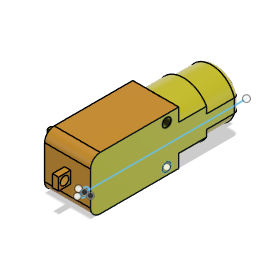
Moto-réducteur (Autodesk Fusion 360 design; units mm, degrees)
Autodesk Fusion 360 part; units mm, degrees
note: some values were not read from the file. Set by a fixed rule: which sketch regions a step uses.
sketch "Sketch1" plane through (0, 0, 0) normal (0, 0, 1) x (1, 0, 0)
  line L0 (0, 0) -> (19, 0)
  line L1 (19, 0) -> (19, 22)
  line L2 (19, 22) -> (0, 22)
  line L3 (0, 22) -> (0, 0)
  line L4 (0, 22) -> (19, 0)
  line L5 (19, 22) -> (0, 0)
  arc A0 (0, 5.4547) -> (19, 5.4547) centre (9.5, 11) ccw
  arc A1 (19, 16.5453) -> (0, 16.5453) centre (9.5, 11) ccw
  dimension "d1" = 19
  dimension "d2" = 22
  constraint horizontal L0
  constraint vertical L1
  constraint horizontal L2
  constraint vertical L3
  constraint coincident L0.start L3.end
  constraint midpoint L4 A0.centre
  constraint tangent L2 A0
  constraint coincident L3 A1.end
  constraint coincident L3 A0.start
  constraint coincident L1 A0.end
  constraint coincident L1 A1.start
  constraint concentric A0 A1
  measures "d1" distance of L0.start L0.end
  measures "d2" distance of L0.start L2.end
extrude "Extrude1" add sketch "Sketch1" along normal blind 36.5
extrude "Extrude2" add sketch "Sketch1" against normal blind 11.5 contours L4 L5 A0 | L3 L4 L5 A0 A1 | L1 L4 L5 A0 A1 | L4 L5 A1
sketch "Sketch2" plane through (0, 0, -11.5) normal (0, 0, -1) x (-1, 0, 0)
  arc A0 (0, 16.5453) -> (-19, 16.5453) centre (-9.5, 11) ccw
  line L0 (-19, 16.5453) -> (-19, 5.4547)
  arc A1 (-19, 5.4547) -> (0, 5.4547) centre (-9.5, 11) ccw
  line L1 (0, 5.4547) -> (0, 16.5453)
  arc A2 (-19, 8.2143) -> (0, 8.2143) centre (-9.5, 11) ccw
  arc A3 (0, 13.7857) -> (-19, 13.7857) centre (-9.5, 11) ccw
  line L2 (-19, 13.7857) -> (-19, 8.2143)
  line L3 (0, 13.7857) -> (0, 8.2143)
  dimension "d7" = 19.8
  constraint concentric A0 A2
  constraint coincident L0 A3.end
  constraint coincident L0 A2.start
  constraint coincident L1 A2.end
  constraint coincident L1 A3.start
  constraint concentric A2 A3
  measures "d7" diameter of A2
extrude "Extrude3" add sketch "Sketch2" along normal blind 13.5 contours L0 L1 A2 A3 L2 L3
sketch "Sketch3" plane through (0, 0, 0) normal (-1, 0, 0) x (0, 0, 1)
  line L0 (0, 22) -> (0, 16.5453)
  line L1 (0, 16.5453) -> (-11.5, 16.5453)
  line L2 (-11.5, 16.5453) -> (-11.5, 13.7857)
  line L3 (-11.5, 13.7857) -> (-25, 13.7857)
  line L4 (-25, 13.7857) -> (-25, 8.2143)
  line L5 (-25, 8.2143) -> (-11.5, 8.2143)
  line L6 (-11.5, 8.2143) -> (-11.5, 5.4547)
  line L7 (-11.5, 5.4547) -> (0, 5.4547)
  line L8 (0, 5.4547) -> (0, 0)
  line L9 (0, 0) -> (36.5, 0)
  line L10 (36.5, 0) -> (36.5, 22)
  line L11 (36.5, 22) -> (0, 22)
  line L12 (36.5, 0) -> (14.5, 0)
  line L13 (14.5, 0) -> (14.5, 22)
  line L14 (14.5, 22) -> (36.5, 22)
  line L15 (36.5, 22) -> (36.5, 0)
  line L16 (14.5, 22) -> (36.5, 0)
  line L17 (36.5, 22) -> (14.5, 0)
  line L18 (24.625, 8.6581) -> (24.625, 13.3419)
  line L19 (26.375, 13.3419) -> (26.375, 8.6581)
  line L20 (26.375, 8.6581) -> (24.625, 13.3419) construction
  line L21 (24.625, 8.6581) -> (26.375, 13.3419) construction
  arc A0 (24.625, 8.6581) -> (26.375, 8.6581) centre (25.5, 11) ccw
  arc A1 (26.375, 13.3419) -> (24.625, 13.3419) centre (25.5, 11) ccw
  circle A2 centre (25.5, 11) radius 2.75
  circle A3 centre (25.5, 11) radius 3
  point P0 (25.5, 11)
  dimension "d10" = 22
  dimension "d11" = 22
  dimension "d12" = 5
  dimension "d13" = 1.75
  dimension "d39" = 5.5
  dimension "d40" = 6
  constraint horizontal L12
  constraint vertical L13
  constraint horizontal L14
  constraint vertical L15
  constraint coincident L9.end L10.start
  constraint coincident L10.end L11.start
  constraint midpoint L16 P0
  constraint parallel L18 L19
  constraint coincident L20 P0
  constraint coincident L21 P0
  constraint coincident P0 A0.centre
  constraint concentric A0 A1
  constraint concentric A0 A2
  measures "d10" distance of L9.end L12.end
  measures "d11" distance of L9.end L10.end
  measures "d12" diameter of A0
  measures "d13" distance of L18.end L19.start
  measures "d39" diameter of A2
  measures "d40" diameter of A3
sketch "Sketch4" plane through (0, 0, -25) normal (0, 0, -1) x (-1, 0, 0)
  line L0 (-19, 13.7857) -> (-19, 8.2143)
  arc A0 (-19, 8.2143) -> (0, 8.2143) centre (-9.5, 11) ccw
  line L1 (0, 8.2143) -> (0, 13.7857)
  arc A1 (0, 13.7857) -> (-19, 13.7857) centre (-9.5, 11) ccw
  circle A2 centre (-9.5, 11) radius 4.75
  dimension "d14" = 9.5
  constraint concentric A0 A2
  measures "d14" diameter of A2
extrude "Extrude4" add sketch "Sketch4" along normal blind 2.5 contours A2
extrude "Extrude5" add sketch "Sketch3" along normal blind 9 contours L16 L17 L18 L19 A1 | L16 L17 L18 | L16 L17 L19 | L16 L17 L18 L19 A0
sketch "Sketch5" plane through (0, 0, 36.5) normal (0, 0, 1) x (1, 0, 0)
  line L0 (0, 22) -> (0, 0)
  line L1 (0, 0) -> (19, 0)
  line L2 (19, 0) -> (19, 22)
  line L3 (19, 22) -> (0, 22)
  line L4 (0, 22) -> (19, 0)
  line L5 (10.75, 13.5) -> (8.25, 13.5)
  line L6 (8.25, 13.5) -> (8.25, 8.5)
  line L7 (8.25, 8.5) -> (10.75, 8.5)
  line L8 (10.75, 8.5) -> (10.75, 13.5)
  line L9 (10.75, 13.5) -> (8.25, 8.5) construction
  line L10 (8.25, 13.5) -> (10.75, 8.5) construction
  point P0 (9.5, 11)
  dimension "d19" = 2.5
  dimension "d20" = 5
  constraint coincident L0.start L3.end
  constraint coincident L1.end L2.start
  constraint horizontal L5
  constraint perpendicular L5 L6
  constraint parallel L5 L7
  constraint parallel L6 L8
  constraint coincident L9 P0
  constraint coincident L10 P0
  constraint midpoint L4 P0
  measures "d19" distance of L6.end L7.end
  measures "d20" distance of L5.end L6.end
extrude "Extrude6" add sketch "Sketch5" along normal blind 5 contours L4 L5 L6 L8 | L4 L6 L7 L8
sketch "Sketch6" plane through (0, 0, -27.5) normal (0, 0, -1) x (-1, 0, 0)
  circle A0 centre (-9.5, 11) radius 4.75
  circle A1 centre (-9.5, 11) radius 0.9
  dimension "d23" = 1.8
  constraint concentric A0 A1
  measures "d23" diameter of A1
extrude "Extrude7" add sketch "Sketch6" along normal blind 0.1 contours A1
fillet "Fillet1" radius 0.9 1 edges at (10.3391, 10.6745, -27.6)
fillet "Fillet2" radius 2 4 edges at (9.5, 20.9, -25) (9.5, 1.1, -25) (19, 11, -25) (0, 11, -25)
fillet "Fillet3" radius 4 2 edges at (9.5, 22, 36.5) (9.5, 0, 36.5)
sketch "Sketch7" plane through (19, 0, 0) normal (1, 0, 0) x (0, 0, -1)
  arc A0 (-36.5, 4) -> (-32.5, 0) centre (-32.5, 4) ccw
  line L0 (-32.5, 0) -> (0, 0)
  line L1 (0, 0) -> (0, 5.4547)
  line L2 (0, 5.4547) -> (11.5, 5.4547)
  line L3 (11.5, 5.4547) -> (11.5, 8.2143)
  line L4 (11.5, 8.2143) -> (23, 8.2143)
  line L5 (23, 8.2143) -> (23, 13.7857)
  line L6 (23, 13.7857) -> (11.5, 13.7857)
  line L7 (11.5, 13.7857) -> (11.5, 16.5453)
  line L8 (11.5, 16.5453) -> (0, 16.5453)
  line L9 (0, 16.5453) -> (0, 22)
  line L10 (0, 22) -> (-32.5, 22)
  arc A1 (-32.5, 22) -> (-36.5, 18) centre (-32.5, 18) ccw
  line L11 (-36.5, 18) -> (-36.5, 4)
  circle A2 centre (-5, 19) radius 1.75
  line L12 (-42, 11) -> (28, 11)
  circle A3 centre (-5, 3) radius 1.75
  line L13 (-41.5, 13.5) -> (-36.5, 8.4999)
  circle A4 centre (-39, 10.9999) radius 1.75
  dimension "d32" = 3.5
  dimension "d33" = 3
  dimension "d34" = 5
  dimension "d38" = 3.5
  constraint perpendicular L5 L12
  constraint symmetric A2 L12 A3
  constraint coincident L11 L13.end
  constraint midpoint L13 A4.centre
  measures "d32" diameter of A2
  measures "d33" distance of L10 A2.centre
  measures "d34" distance of L9 A2.centre
  measures "d38" diameter of A4
extrude "Extrude8" cut sketch "Sketch7" against normal blind 20 contours L12 L13 A4 | L12 L13 A4 | L12 L13 A4 | L12 L13 A4 | A2 | A3
extrude "Extrude9" cut sketch "Sketch3" against normal blind 18 contours L16 L17 A2 A3 | L16 L17 A2 A3 | L16 L17 A2 A3 | L16 L17 A2 A3
